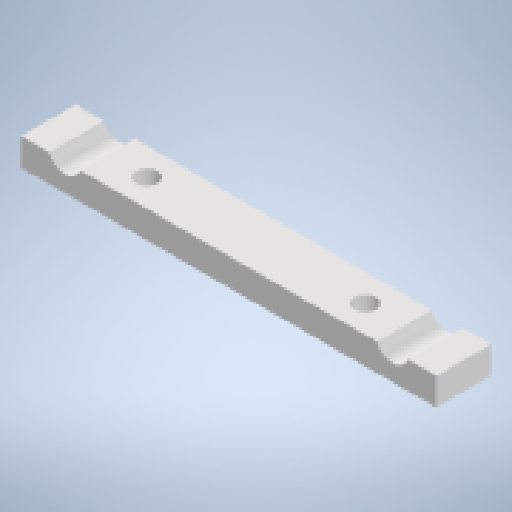
# Autodesk Inventor part: 6_2xclamp_back
Saved by Autodesk Inventor 2025.1 (Build 291241000, 241)
## iProperties
Created: 2024-10-31
Part Number: 6_2xclamp_back
Material: Ogólny
Document SubType Name: Modeling
Designer: PC
Density: 1 g/cm^3
Appearance: Domyślna
Author: PC
Autodesk Inventor part; units mm, degrees
ref_plane "YZ Plane" through (0, 0, 0) normal (1, 0, 0) x (0, 1, 0)
ref_plane "XZ Plane" through (0, 0, 0) normal (0, 1, 0) x (-1, 0, 0)
sketch "Szkic1" plane through (0, 0, 0) normal (0, 0, 1) x (1, 0, 0)
  arc A0 (33, -4) -> (27, -4) centre (30, -4) ccw projected
  arc A1 (-27, -4) -> (-33, -4) centre (-30, -4) ccw projected
  circle A2 centre (30, -4) radius 3 construction
  circle A3 centre (-30, -4) radius 3 construction
  line L0 (-38, -5) -> (-38, -10)
  line L1 (-38, -10) -> (38, -10)
  line L2 (38, -10) -> (38, -5)
  line L3 (-38, 2) -> (-38, -4) construction
  line L4 (38, -4) -> (38, 2) construction
  arc A4 (27.1716, -5) -> (32.8284, -5) centre (30, -4) ccw
  arc A5 (-32.8284, -5) -> (-27.1716, -5) centre (-30, -4) ccw
  line L5 (-32.8284, -5) -> (-38, -5)
  line L6 (38, -5) -> (32.8284, -5)
  line L7 (27.1716, -5) -> (-27.1716, -5)
  point P0 (0, 0)
  dimension "d1" = 5
  constraints: 12 end point, 4 centre point, 4 coincident, 4 parallel, 4 point on circle, 3 horizontal, 3 perpendicular, 2 collinear, 2 concentric
  measures "d1" distance of L1.end L2.end
ref_plane "Płaszczyzna konstrukcyjna1" through (-38, -4, -10) normal (0, 0, -1) x (0, 1, 0)
extrude "Wyciągnięcie proste1" add sketch "Szkic1" against normal up to surface (10 mm away)
sketch "Szkic2" plane through (-38, -10, 0) normal (0, -1, 0) x (1, 0, 0)
  circle A0 centre (58, -5) radius 1.75 projected
  circle A1 centre (18, -5) radius 1.75 projected
  circle A2 centre (58, -5) radius 2
  circle A3 centre (18, -5) radius 2
  point P0 (38, 0)
  dimension "d4" = 4
  dimension "d5" = 4
  constraints: 2 centre point, 2 coincident
  measures "d4" diameter of A2
  measures "d5" diameter of A3
extrude "Wyciągnięcie proste2" cut sketch "Szkic2" against normal up to next contours A0 | A1 | A2 | A3
